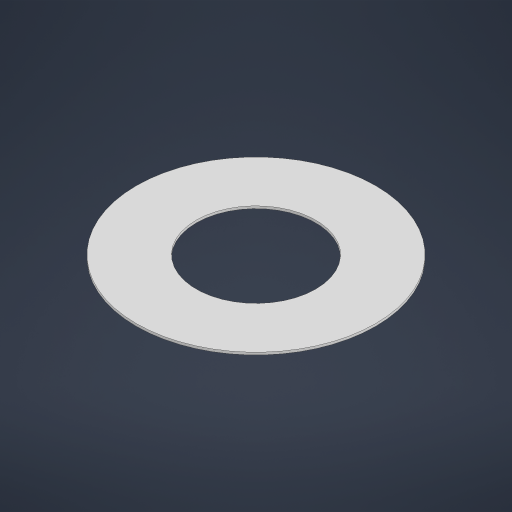
# Autodesk Inventor part: m10 washa
Saved by Autodesk Inventor 2024 (Build 280153000, 153)
## iProperties
Created: 2023-06-18
Part Number: m10 washa
Material: 일반
Document SubType Name: Modeling
Designer: 6gioc
Density: 1 g/cm^3
Appearance: 기본값
Author: 6gioc
## iProperties of the stored document m10 washa_3D 인쇄.ipt
Created: 2023-06-20
Part Number: m10 washa_3D 인쇄
Material: 일반
Document SubType Name: Modeling
Designer: 6gioc
Density: 1 g/cm^3
Appearance: 기본값
Author: 6gioc
Autodesk Inventor part; units mm, degrees
ref_plane "YZ Plane" through (0, 0, 0) normal (1, 0, 0) x (0, 1, 0)
ref_plane "XZ Plane" through (0, 0, 0) normal (0, 1, 0) x (-1, 0, 0)
ref_plane "XY Plane" through (0, 0, 0) normal (0, 0, 1) x (1, 0, 0)
sketch "스케치1" plane through (0, 0, 0) normal (0, 1, 0) x (-1, 0, 0)
  circle A0 centre (0, 0) radius 5
  circle A1 centre (0, 0) radius 10
  dimension "d0" = 10
  dimension "d1" = 20
  constraints: 2 centre point, 2 coincident
  measures "d0" diameter of A0
  measures "d1" diameter of A1
extrude "돌출1" add sketch "스케치1" along normal blind 0.2
